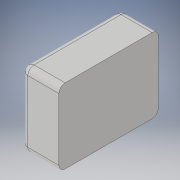
# Autodesk Inventor part: electronicsbay
Saved by Autodesk Inventor 2018 (Build 220112000, 112)
## iProperties
Created: 2020-03-14
Part Number: electronicsbay
Material: Generic
Document SubType Name: Modeling
Designer: natha
Density: 1 g/cm^3
Appearance: Default
Author: natha
Autodesk Inventor part; units mm, degrees
ref_plane "YZ Plane" through (0, 0, 0) normal (1, 0, 0) x (0, 1, 0)
ref_plane "XZ Plane" through (0, 0, 0) normal (0, 1, 0) x (-1, 0, 0)
ref_plane "XY Plane" through (0, 0, 0) normal (0, 0, 1) x (1, 0, 0)
sketch "Sketch1" plane through (0, 0, 0) normal (0, 1, 0) x (-1, 0, 0)
  line L0 (0, 0) -> (76.2, 0)
  line L1 (76.2, 0) -> (76.2, -203.2)
  line L2 (76.2, -203.2) -> (0, -203.2)
  line L3 (0, -203.2) -> (0, 0)
  dimension "d0" = 76.2
  dimension "d1" = 203.2
  constraints: 8 end point, 2 parallel, 1 horizontal, 1 perpendicular
  measures "d0" distance of L1.end L2.end
  measures "d1" distance of L0.end L1.end
extrude "Extrusion1" add sketch "Sketch1" along normal blind 152.4
fillet "Fillet1" radius 12.7 8 edges at (-38.1, 152.4, 0) (-38.1, 0, 0) (-76.2, 76.2, 0) (-76.2, 152.4, -101.6) (-38.1, 152.4, -203.2) (-38.1, 0, -203.2) (-76.2, 76.2, -203.2) (-76.2, 0, -101.6)
body "Solid1"
